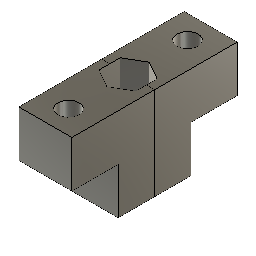
module_stand (Autodesk Fusion 360 design; units mm, degrees)
Autodesk Fusion 360 part; units mm, degrees
sketch "Skizze1" plane through (0, 0, 0) normal (1, 0, 0) x (0, 1, 0)
  line L0 (0, 0) -> (0, 14)
  line L1 (0, 14) -> (12.5, 14)
  line L2 (12.5, 14) -> (12.5, 7)
  line L3 (12.5, 7) -> (5.5, 7)
  line L4 (5.5, 7) -> (5.5, 0)
  line L5 (5.5, 0) -> (0, 0)
  dimension "d1" = 5.5
  dimension "d2" = 7
  dimension "d3" = 14
  dimension "d4" = 12.5
  constraint coincident L0.start L5.end
  constraint vertical L0
  constraint perpendicular L0 L1
  constraint perpendicular L1 L2
  constraint perpendicular L2 L3
  constraint perpendicular L1 L4
  constraint perpendicular L4 L5
  measures "d1" distance of L0.start L4.end
  measures "d2" distance of L3.end L4.end
  measures "d3" distance of L0.start L0.end
  measures "d4" distance of L0.end L1.end
extrude "Extrusion1" add sketch "Skizze1" along normal blind 8 makes body 1
sketch "Skizze2" plane through (0, 0, 14) normal (0, 0, 1) x (-1, 0, 0)
  line L0 (0, -12.5) -> (0, 0)
  line L1 (0, 0) -> (-8, 0)
  line L2 (-8, 0) -> (-8, -12.5)
  line L3 (-8, -12.5) -> (0, -12.5)
  point P0 (-4, 0)
  point P1 (-4, -9)
  dimension "d7" = 4
  dimension "d8" = 4
  dimension "d10" = 3.5
  constraint coincident L1 P0
  measures "d7" distance of L2 P1
  measures "d8" distance of L2 P0
  measures "d10" distance of L3 P1
hole "Bohrung1" at (4, 0, 14) at (4, 9, 14) direction (0, 0, -1) diameter 3.2 end through all bodies 1
sketch "Skizze3" plane through (0, 0, 14) normal (0, 0, 1) x (-1, 0, 0)
  arc A0 (-5.6, 0) -> (-2.4, 0) centre (-4, 0) ccw
  line L0 (-5.6, 0) -> (-8, 0)
  line L1 (-8, 0) -> (-8, -12.5)
  line L2 (-8, -12.5) -> (0, -12.5)
  line L3 (0, -12.5) -> (0, 0)
  line L4 (0, 0) -> (-2.4, 0)
  circle A1 centre (-4, -9) radius 1.6
  line L5 (-1.2, 1.6166) -> (-4, 3.2332)
  line L6 (-4, 3.2332) -> (-6.8, 1.6166)
  line L7 (-6.8, 1.6166) -> (-6.8, -1.6166)
  line L8 (-6.8, -1.6166) -> (-4, -3.2332)
  line L9 (-4, -3.2332) -> (-1.2, -1.6166)
  line L10 (-1.2, -1.6166) -> (-1.2, 1.6166)
  point P0 (-4, 0)
  dimension "d14" = 5.6
  constraint coincident P0 A0.centre
  constraint parallel L1 L7
  measures "d14" distance of L7 L10
extrude "Extrusion2" cut sketch "Skizze3" against normal blind 7 contours A0 L0 L4 L7 L8 L9 L10 bodies 1
sketch "Skizze4" plane through (0, 0, 7) normal (0, 0, -1) x (1, 0, 0)
  circle A0 centre (4, -9) radius 1.6
  line L0 (0, -5.5) -> (0, -12.5)
  line L1 (0, -12.5) -> (8, -12.5)
  line L2 (8, -12.5) -> (8, -5.5)
  line L3 (8, -5.5) -> (0, -5.5)
  line L4 (6.8, -7.3834) -> (4, -5.7668)
  line L5 (4, -5.7668) -> (1.2, -7.3834)
  line L6 (1.2, -7.3834) -> (1.2, -10.6166)
  line L7 (1.2, -10.6166) -> (4, -12.2332)
  line L8 (4, -12.2332) -> (6.8, -10.6166)
  line L9 (6.8, -10.6166) -> (6.8, -7.3834)
  point P0 (4, -9)
  dimension "d17" = 5.6
  constraint coincident P0 A0.centre
  constraint parallel L0 L6
  measures "d17" distance of L6 L9
extrude "Extrusion3" cut sketch "Skizze4" against normal blind 4 contours L4 L5 L6 L7 L8 L9 bodies 1
mirror "Spiegeln1" about plane through (0, 0, 0) normal (0, -1, 0) of "Extrusion1", "Bohrung1", "Extrusion2", "Extrusion3" makes body 2
equation "d1 = ( 11 / 2 ) * 1 mm"
equation "d4 = ( 25 / 2 ) * 1 mm"
